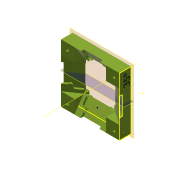
# Autodesk Inventor part: 30_Z_Stage_Fluomodule
Saved by Autodesk Inventor 2019 (Build 230136000, 136)
## iProperties
Created: 2019-07-09
Part Number: 30_Z_Stage_Fluomodule
Material: Generic
Document SubType Name: Modeling
Designer: diederichbenedict
Density: 1 g/cm^3
Appearance: IPHT_Türkis
Author: diederichbenedict
Autodesk Inventor part; units mm, degrees
ref_plane "Work Plane1" through (0, 0, 10) normal (0, 0, 1) x (1, 0, 0)
sketch "Sketch1" plane through (0, 0, 10) normal (0, 0, 1) x (1, 0, 0)
  circle A0 centre (0, 0) radius 15 construction
  circle A1 centre (-19.9, -20) radius 1.5 projected
  circle A2 centre (20.1, -20) radius 1.5 projected
  circle A3 centre (20.1, 19.85) radius 1.5 projected
  circle A4 centre (-19.9, 19.85) radius 1.5 projected
  line L0 (-25, 25) -> (25, 25) construction
  line L1 (-25, -25) -> (-25, 25) construction
  line L2 (25, -25) -> (-25, -25) construction
  line L3 (25, 25) -> (25, -25) construction
  line L4 (25, 25) -> (-25, 25)
  line L5 (-25, 25) -> (-25, -25)
  line L6 (-25, -25) -> (25, -25)
  line L7 (25, -25) -> (25, 25)
  circle A5 centre (0, 0) radius 15
  circle A6 centre (0, 0) radius 13
  point P0 (0, 0)
  dimension "d15" = 2
  constraints: 8 end point, 2 centre point, 2 parallel, 1 coincident, 1 concentric, 1 horizontal, 1 perpendicular
  measures "d15" radial gap between concentric circles of A0 A6
extrude "Extrusion1" add sketch "Sketch1" along normal blind 10 contours L7 L6 L5 L4 | A5
ref_plane "Work Plane2" through (-25, 0, 10) normal (0, -1, 0) x (1, 0, 0)
ref_plane "Work Plane3" through (-24.8, 13.5, 23.5) normal (0, -1, 0) x (1, 0, 0)
ref_plane "Work Plane4" through (-24.8, -13.5, 23.5) normal (0, 1, 0) x (0, 0, 1)
ref_plane "Work Plane5" through (-24.8, 13.5, 25.5) normal (0, -1, 0) x (1, 0, 0)
ref_plane "Work Plane6" through (-24.8, -13.5, 25.5) normal (0, 1, 0) x (0, 0, 1)
sketch "Sketch2" plane through (-25, 0, 10) normal (0, -1, 0) x (1, 0, 0)
  line L0 (50, 10) -> (0, 10) projected
  line L1 (10, 10) -> (40, 10) projected
  line L2 (0, 0) -> (0, 10) projected
  line L3 (0, 10) -> (25, -7.5052)
  line L4 (0, 10) -> (30.5194, 10) construction
  line L5 (25, -7.5052) -> (25, 10)
  line L6 (0, 10) -> (25, 10)
  point P0 (25, -10)
  point P1 (22.6369, 10)
  dimension "d8" = 35
  constraints: 8 end point, 1 collinear, 1 equal length, 1 horizontal, 1 midpoint, 1 point on line
  measures "d8" angle of L3 L4
extrude "Extrusion2" cut sketch "Sketch2" along normal up to surface (27 mm away) from surface at -13.5
pattern_circular "Circular Pattern1" count 4 over 360 about axis through (0, 0, 10) along (0, 0, 1) of "Extrusion2"
sketch "Sketch3" plane through (-13.5, -25, 20) normal (0, 0.5736, 0.8192) x (1, 0, 0)
  line L0 (-11.5, 5.7358) -> (38.5, 5.7358) projected
  circle A0 centre (13.5, 10.7656) radius 4.6099 construction
  point P0 (13.5, 31.9503)
  constraints: 1 centre point
sketch "Sketch4" plane through (-13.5, -13.5, 11.9476) normal (0, 0.5736, 0.8192) x (1, 0, 0)
  arc A0 (20.4949, 3.7045) -> (20.3821, 4.3003) centre (20.1821, 3.9539) ccw construction
  arc A1 (20.4949, 3.7045) -> (23.0404, -0.7044) centre (22.6326, 1.9994) ccw construction
  arc A2 (23.5, -1.0999) -> (23.0404, -0.7044) centre (23.1, -1.0999) ccw construction
  line L0 (23.5, -5.4466) -> (23.5, -1.0999) construction
  arc A3 (23.0404, -5.8421) -> (23.5, -5.4466) centre (23.1, -5.4466) ccw construction
  arc A4 (23.0404, -5.8421) -> (20.4949, -10.251) centre (22.6326, -8.546) ccw construction
  arc A5 (20.3821, -10.8469) -> (20.4949, -10.251) centre (20.1821, -10.5004) ccw construction
  line L1 (16.6179, -13.0202) -> (20.3821, -10.8469) construction
  arc A6 (16.0455, -12.8199) -> (16.6179, -13.0202) centre (16.4179, -12.6738) ccw construction
  arc A7 (16.0455, -12.8199) -> (10.9545, -12.8199) centre (13.5, -13.8187) ccw construction
  arc A8 (10.3821, -13.0202) -> (10.9545, -12.8199) centre (10.5821, -12.6738) ccw construction
  line L2 (6.6179, -10.8469) -> (10.3821, -13.0202) construction
  arc A9 (6.5051, -10.251) -> (6.6179, -10.8469) centre (6.8179, -10.5004) ccw construction
  arc A10 (6.5051, -10.251) -> (3.9596, -5.8421) centre (4.3674, -8.546) ccw construction
  arc A11 (3.5, -5.4466) -> (3.9596, -5.8421) centre (3.9, -5.4466) ccw construction
  line L3 (3.5, -1.0999) -> (3.5, -5.4466) construction
  arc A12 (3.9596, -0.7044) -> (3.5, -1.0999) centre (3.9, -1.0999) ccw construction
  arc A13 (3.9596, -0.7044) -> (6.5051, 3.7045) centre (4.3674, 1.9994) ccw construction
  arc A14 (6.6179, 4.3003) -> (6.5051, 3.7045) centre (6.8179, 3.9539) ccw construction
  line L4 (10.3821, 6.4736) -> (6.6179, 4.3003) construction
  arc A15 (10.9545, 6.2733) -> (10.3821, 6.4736) centre (10.5821, 6.1272) ccw construction
  arc A16 (10.9545, 6.2733) -> (16.0455, 6.2733) centre (13.5, 7.2721) ccw construction
  arc A17 (16.6179, 6.4736) -> (16.0455, 6.2733) centre (16.4179, 6.1272) ccw construction
  line L5 (20.3821, 4.3003) -> (16.6179, 6.4736) construction
  arc A18 (17.1179, 7.3397) -> (15.1146, 6.6386) centre (16.4179, 6.1272) ccw
  arc A19 (11.8854, 6.6386) -> (15.1146, 6.6386) centre (13.5, 7.2721) ccw
  arc A20 (11.8854, 6.6386) -> (9.8821, 7.3397) centre (10.5821, 6.1272) ccw
  line L6 (9.8821, 7.3397) -> (6.1179, 5.1664)
  arc A21 (6.1179, 5.1664) -> (5.7234, 3.081) centre (6.8179, 3.9539) ccw
  arc A22 (4.1088, 0.2844) -> (5.7234, 3.081) centre (4.3674, 1.9994) ccw
  arc A23 (4.1088, 0.2844) -> (2.5, -1.0999) centre (3.9, -1.0999) ccw
  line L7 (2.5, -1.0999) -> (2.5, -5.4466)
  arc A24 (2.5, -5.4466) -> (4.1088, -6.8309) centre (3.9, -5.4466) ccw
  arc A25 (5.7234, -9.6275) -> (4.1088, -6.8309) centre (4.3674, -8.546) ccw
  arc A26 (5.7234, -9.6275) -> (6.1179, -11.7129) centre (6.8179, -10.5004) ccw
  line L8 (6.1179, -11.7129) -> (9.8821, -13.8862)
  arc A27 (9.8821, -13.8862) -> (11.8854, -13.1851) centre (10.5821, -12.6738) ccw
  arc A28 (15.1146, -13.1851) -> (11.8854, -13.1851) centre (13.5, -13.8187) ccw
  arc A29 (15.1146, -13.1851) -> (17.1179, -13.8862) centre (16.4179, -12.6738) ccw
  line L9 (17.1179, -13.8862) -> (20.8821, -11.7129)
  arc A30 (20.8821, -11.7129) -> (21.2766, -9.6275) centre (20.1821, -10.5004) ccw
  arc A31 (22.8912, -6.8309) -> (21.2766, -9.6275) centre (22.6326, -8.546) ccw
  arc A32 (22.8912, -6.8309) -> (24.5, -5.4466) centre (23.1, -5.4466) ccw
  line L10 (24.5, -5.4466) -> (24.5, -1.0999)
  arc A33 (24.5, -1.0999) -> (22.8912, 0.2844) centre (23.1, -1.0999) ccw
  arc A34 (21.2766, 3.081) -> (22.8912, 0.2844) centre (22.6326, 1.9994) ccw
  arc A35 (21.2766, 3.081) -> (20.8821, 5.1664) centre (20.1821, 3.9539) ccw
  line L11 (20.8821, 5.1664) -> (17.1179, 7.3397)
  line L12 (21.5577, -10.7607) -> (5.4423, -10.7607)
  line L13 (5.4423, -10.7607) -> (5.4423, -14.6808)
  line L14 (5.4423, -14.6808) -> (21.5577, -14.6808)
  line L15 (21.5577, -14.6808) -> (21.5577, -10.7607)
  point P0 (13.5, 17.9114)
  dimension "d16" = 1
  constraints: 37 point on circle, 20 end point, 18 centre point, 2 parallel, 1 horizontal, 1 perpendicular, 23 other
  measures "d16" distance between parallel lines of L5 L11
extrude "Extrusion4" cut sketch "Sketch4" against normal blind 2
pattern_circular "Circular Pattern3" count 4 over 360 about axis through (0.2, 0, 46.5088) along (0, 0, 1) of "Extrusion4"
sketch "Sketch5" plane through (25, -25, 10) normal (1, 0, 0) x (0, 0, -1)
  line L0 (-7.4184, 32.8577) -> (-7.4184, 16.7423) projected
  line L1 (-7.4184, 16.7423) -> (-9.86, 16.7423) projected
  line L2 (-9.86, 16.7423) -> (-9.86, 32.8577) projected
  line L3 (-9.86, 32.8577) -> (-7.4184, 32.8577) projected
  line L4 (0, 0) -> (0, 50) projected
  line L5 (0, 50) -> (-10, 50) projected
  line L6 (-10, 38.5) -> (-10, 50) projected
  line L7 (-10, 11.5) -> (-10, 38.5) projected
  line L8 (-10, 0) -> (-10, 11.5) projected
  line L9 (0, 0) -> (-10, 0) projected
  line L10 (-6.3859, 36.4329) -> (-6.3859, 47.5514) construction
  line L11 (-6.3859, 47.5514) -> (10.2283, 47.5514) construction
  line L12 (10.2283, 47.5514) -> (10.2283, 36.4329) construction
  line L13 (10.2283, 36.4329) -> (-6.3859, 36.4329) construction
  point P0 (10, 25)
  constraints: 2 other
body "Solid1"
